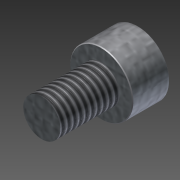
# Autodesk Inventor part: M5_8mm
Saved by Autodesk Inventor 2011 (Build 150239000, 239)
## iProperties
Created: 2013-02-08
Part Number: M5_8mm
Document SubType Name: Modeling
Designer: arihon
Density: 1 g/cm^3
Author: arihon
Autodesk Inventor part; units mm, degrees
ref_plane "YZ Plane" through (0, 0, 0) normal (1, 0, 0) x (0, 1, 0)
ref_plane "XZ Plane" through (0, 0, 0) normal (0, 1, 0) x (-1, 0, 0)
ref_plane "XY Plane" through (0, 0, 0) normal (0, 0, 1) x (1, 0, 0)
sketch "スケッチ1" plane through (0, 0, 0) normal (0, 0, 1) x (1, 0, 0)
  line L0 (-4.25, 5) -> (0, 5)
  line L1 (4.25, 5) -> (4.25, 0)
  line L2 (4.25, 0) -> (-4.25, 0)
  line L3 (-4.25, 0) -> (-4.25, 5)
  line L4 (-2.5, 0) -> (0, 0)
  line L5 (2.5, 0) -> (2.5, -8)
  line L6 (2.5, -8) -> (0, -8)
  line L7 (-2.5, -8) -> (-2.5, 0)
  line L8 (0, 5) -> (0, -8)
  line L9 (0, 5) -> (4.25, 5)
  line L10 (0, 0) -> (2.5, 0)
  line L11 (0, -8) -> (-2.5, -8)
  point P0 (0, 0)
  dimension "d0" = 5
  dimension "d1" = 2.5
  dimension "d2" = 8
  dimension "d3" = 8.5
  dimension "d4" = 4.25
  dimension "d5" = 5
  dimension "d18" = 5
  constraints: 24 end point, 9 parallel, 4 horizontal, 4 perpendicular, 2 point on line
  measures "d0" distance of L5.end L7.start
  measures "d1" distance from line of L5 point (0, 0)
  measures "d2" distance of L5.start L5.end
  measures "d3" distance of L0.start L1.start
  measures "d4" distance from line of L3 point (0, 0)
  measures "d5" distance of L1.start L1.end
  measures "d18" diameter of L5 L8
revolve "回転1" add sketch "スケッチ1" angle 360 about axis through (0, 5, 0) along (0, -1, 0) contours L0 L8 L2 L3 | L8 L11 L7 L2
sketch "スケッチ2" plane through (0, 5, 0) normal (0, 1, 0) x (1, 0, 0)
  line L0 (0, 2.3094) -> (2, 1.1547)
  line L1 (2, 1.1547) -> (2, -1.1547)
  line L2 (2, -1.1547) -> (0, -2.3094)
  line L3 (0, -2.3094) -> (-2, -1.1547)
  line L4 (-2, -1.1547) -> (-2, 1.1547)
  line L5 (-2, 1.1547) -> (0, 2.3094)
  point P0 (0, 0)
  dimension "d9" = 4
  constraints: 12 end point, 13 other
  measures "d9" distance between parallel lines of L3 L0
extrude "押し出し1" cut sketch "スケッチ2" against normal blind 3
chamfer "面取り1" distance 0.1 angle 45 2 edges at (4.25, 5, 0) (4.25, 0, 0)
chamfer "面取り2" distance 0.2 angle 45 6 edges at (1, 5, 1.7321) (-1, 5, 1.7321) (-2, 5, 0) (-1, 5, -1.7321) (1, 5, -1.7321) (2, 5, 0)
thread "ねじ2" size "M5x0.8" class "6g" standard "ANSI Metric M Profile" full length
equation "\"d1\" = 0.5 * d0"
equation "\"d4\" = 0.5 * d3"
equation "\"d18\" = d0"
